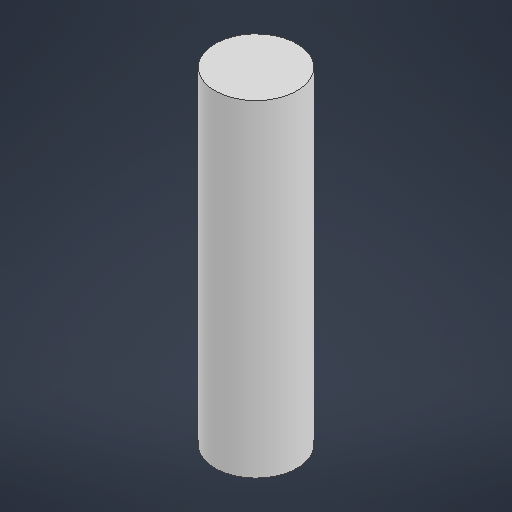
# Autodesk Inventor part: Eixo5
Saved by Autodesk Inventor 2026.2 (Build 302298000, 298)
## iProperties
Created: 2026-09-18
Part Number: Eixo5
Material: Genérico
Document SubType Name: Modeling
Designer: IFSP
Density: 1 g/cm^3
Appearance: Padrão
Author: IFSP
Autodesk Inventor part; units mm, degrees
ref_plane "YZ Plane" through (0, 0, 0) normal (1, 0, 0) x (0, 1, 0)
ref_plane "XZ Plane" through (0, 0, 0) normal (0, 1, 0) x (-1, 0, 0)
ref_plane "XY Plane" through (0, 0, 0) normal (0, 0, 1) x (1, 0, 0)
sketch "Esboço1" plane through (0, 0, 0) normal (0, 1, 0) x (-1, 0, 0)
  circle A0 centre (0, 0) radius 4.765
  dimension "d10" = 9.53
  constraints: 1 centre point
  measures "d10" diameter of A0
extrude "Extrusão1" add sketch "Esboço1" along normal blind 38.1
